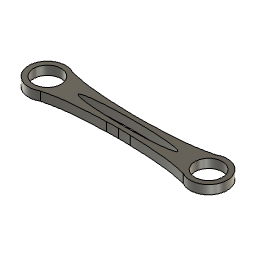
First Arm (Autodesk Fusion 360 design; units mm, degrees)
Autodesk Fusion 360 part; units mm, degrees
note: some values were not read from the file. Set by a fixed rule: which sketch regions a step uses.
sketch "Sketch1" plane through (0, 0, 0) normal (0, 0, 1) x (1, 0, 0)
  circle A0 centre (0, 0) radius 11.0625
  circle A1 centre (0, 0) radius 15
  line L0 (0, 0) -> (130, 0)
  circle A2 centre (130, 0) radius 11.0625
  circle A3 centre (130, 0) radius 15
  line L1 (0, 0) -> (65, 0)
  spline S0 degree 5 poles (7.4528, 13.0175) (7.8836, 12.9141) (8.7411, 12.7102) (10.015, 12.4132) (11.688, 12.0352) (13.7317, 11.594) (15.7226, 11.1861) (17.6579, 10.8135) (19.5392, 10.4779) (21.3761, 10.1803) (23.1841, 9.9205) (24.9799, 9.6971) (26.7778, 9.5065) (28.5855, 9.3432) (30.3994, 9.1985) (32.2092, 9.0627) (34.0044, 8.9273) (35.7794, 8.7866) (37.5401, 8.6406) (39.3083, 8.496) (41.1126, 8.3625) (42.9802, 8.2492) (44.9302, 8.1618) (46.9629, 8.0975) (49.0581, 8.0448) (51.1857, 7.988) (52.8875, 7.9263) (54.152, 7.865) (54.9881, 7.8168) (55.4044, 7.7909) knots 0 0 0 0 0 0 0.04 0.08 0.12 0.16 0.2 0.24 0.28 0.32 0.36 0.4 0.44 0.48 0.52 0.56 0.6 0.64 0.68 0.72 0.76 0.8 0.84 0.88 0.92 0.96 1 1 1 1 1 1
  line L2 (65, 0) -> (65, 43.1808)
  spline S1 degree 5 poles (55.4044, 7.7909) (55.7874, 7.7593) (56.5538, 7.7035) (57.7049, 7.642) (59.2419, 7.5975) (61.1644, 7.58) (62.701, 7.5793) (63.8515, 7.5799) (64.6173, 7.5801) (65, 7.5801) knots 0 0 0 0 0 0 0.2 0.4 0.6 0.8 1 1 1 1 1 1
  spline S2 degree 5 poles (122.5472, 13.0175) (122.1164, 12.9141) (121.2589, 12.7102) (119.985, 12.4132) (118.312, 12.0352) (116.2683, 11.594) (114.2774, 11.1861) (112.3421, 10.8135) (110.4608, 10.4779) (108.6239, 10.1803) (106.8159, 9.9205) (105.0201, 9.6971) (103.2222, 9.5065) (101.4145, 9.3432) (99.6006, 9.1985) (97.7908, 9.0627) (95.9956, 8.9273) (94.2206, 8.7866) (92.4599, 8.6406) (90.6917, 8.496) (88.8874, 8.3625) (87.0198, 8.2492) (85.0698, 8.1618) (83.0371, 8.0975) (80.9419, 8.0448) (78.8143, 7.988) (77.1125, 7.9263) (75.848, 7.865) (75.0119, 7.8168) (74.5956, 7.7909) knots 0 0 0 0 0 0 0.04 0.08 0.12 0.16 0.2 0.24 0.28 0.32 0.36 0.4 0.44 0.48 0.52 0.56 0.6 0.64 0.68 0.72 0.76 0.8 0.84 0.88 0.92 0.96 1 1 1 1 1 1
  line L3 (2.3089, 14.2524) -> (12.5967, 11.7826)
  line L4 (50.4549, 8.0994) -> (60.354, 7.4823)
  line L5 (127.6911, 14.2524) -> (117.4033, 11.7826)
  line L6 (79.5451, 8.0994) -> (69.646, 7.4823)
  spline S3 degree 5 poles (74.5956, 7.7909) (74.2126, 7.7593) (73.4462, 7.7035) (72.2951, 7.642) (70.7581, 7.5975) (68.8356, 7.58) (67.299, 7.5793) (66.1485, 7.5799) (65.3827, 7.5801) (65, 7.5801) knots 0 0 0 0 0 0 0.2 0.4 0.6 0.8 1 1 1 1 1 1
  line L7 (54.4257, 7.8715) -> (56.3832, 7.7102)
  line L8 (64.0213, 7.5801) -> (65.9787, 7.5801)
  line L9 (75.5743, 7.8715) -> (73.6168, 7.7102)
  line L10 (65.9787, 7.5801) -> (64.0213, 7.5801)
  spline S4 degree 5 poles (122.5472, -13.0175) (122.1164, -12.9141) (121.2589, -12.7102) (119.985, -12.4132) (118.312, -12.0352) (116.2683, -11.594) (114.2774, -11.1861) (112.3421, -10.8135) (110.4608, -10.4779) (108.6239, -10.1803) (106.8159, -9.9205) (105.0201, -9.6971) (103.2222, -9.5065) (101.4145, -9.3432) (99.6006, -9.1985) (97.7908, -9.0627) (95.9956, -8.9273) (94.2206, -8.7866) (92.4599, -8.6406) (90.6917, -8.496) (88.8874, -8.3625) (87.0198, -8.2492) (85.0698, -8.1618) (83.0371, -8.0975) (80.9419, -8.0448) (78.8143, -7.988) (77.1125, -7.9263) (75.848, -7.865) (75.0119, -7.8168) (74.5956, -7.7909) knots 0 0 0 0 0 0 0.04 0.08 0.12 0.16 0.2 0.24 0.28 0.32 0.36 0.4 0.44 0.48 0.52 0.56 0.6 0.64 0.68 0.72 0.76 0.8 0.84 0.88 0.92 0.96 1 1 1 1 1 1
  line L11 (127.6911, -14.2524) -> (117.4033, -11.7826)
  line L12 (79.5451, -8.0994) -> (69.646, -7.4823)
  spline S5 degree 5 poles (74.5956, -7.7909) (74.2126, -7.7593) (73.4462, -7.7035) (72.2951, -7.642) (70.7581, -7.5975) (68.8356, -7.58) (67.299, -7.5793) (66.1485, -7.5799) (65.3827, -7.5801) (65, -7.5801) knots 0 0 0 0 0 0 0.2 0.4 0.6 0.8 1 1 1 1 1 1
  line L13 (75.5743, -7.8715) -> (73.6168, -7.7102)
  line L14 (65.9787, -7.5801) -> (64.0213, -7.5801)
  spline S6 degree 5 poles (55.4044, -7.7909) (55.7874, -7.7593) (56.5538, -7.7035) (57.7049, -7.642) (59.2419, -7.5975) (61.1644, -7.58) (62.701, -7.5793) (63.8515, -7.5799) (64.6173, -7.5801) (65, -7.5801) knots 0 0 0 0 0 0 0.2 0.4 0.6 0.8 1 1 1 1 1 1
  line L15 (54.4257, -7.8715) -> (56.3832, -7.7102)
  line L16 (64.0213, -7.5801) -> (65.9787, -7.5801)
  spline S7 degree 5 poles (7.4528, -13.0175) (7.8836, -12.9141) (8.7411, -12.7102) (10.015, -12.4132) (11.688, -12.0352) (13.7317, -11.594) (15.7226, -11.1861) (17.6579, -10.8135) (19.5392, -10.4779) (21.3761, -10.1803) (23.1841, -9.9205) (24.9799, -9.6971) (26.7778, -9.5065) (28.5855, -9.3432) (30.3994, -9.1985) (32.2092, -9.0627) (34.0044, -8.9273) (35.7794, -8.7866) (37.5401, -8.6406) (39.3083, -8.496) (41.1126, -8.3625) (42.9802, -8.2492) (44.9302, -8.1618) (46.9629, -8.0975) (49.0581, -8.0448) (51.1857, -7.988) (52.8875, -7.9263) (54.152, -7.865) (54.9881, -7.8168) (55.4044, -7.7909) knots 0 0 0 0 0 0 0.04 0.08 0.12 0.16 0.2 0.24 0.28 0.32 0.36 0.4 0.44 0.48 0.52 0.56 0.6 0.64 0.68 0.72 0.76 0.8 0.84 0.88 0.92 0.96 1 1 1 1 1 1
  line L17 (2.3089, -14.2524) -> (12.5967, -11.7826)
  line L18 (50.4549, -8.0994) -> (60.354, -7.4823)
  ellipse E0 centre (65, 0) end of major axis (25, 0) minor radius 4
  line L19 (105, 0) -> (25, 0) construction
  line L20 (65, 4) -> (65, -4) construction
  point P0 (18.3178, 10.6996)
  point P1 (27.044, 9.4876)
  point P2 (35.5289, 8.8053)
  point P3 (44.207, 8.1979)
  point P4 (111.6822, 10.6996)
  point P5 (102.956, 9.4876)
  point P6 (94.4711, 8.8053)
  point P7 (85.793, 8.1979)
  point P8 (111.6822, -10.6996)
  point P9 (102.956, -9.4876)
  point P10 (94.4711, -8.8053)
  point P11 (85.793, -8.1979)
  point P12 (18.3178, -10.6996)
  point P13 (27.044, -9.4876)
  point P14 (35.5289, -8.8053)
  point P15 (44.207, -8.1979)
  dimension "d1" = 22.125
  dimension "d2" = 30
  dimension "d3" = 130
  dimension "d4" = 22.125
  dimension "d5" = 30
  dimension "d6" = 65
  constraint coincident A0.centre A1.centre
  constraint concentric A0 A1
  constraint horizontal L0
  constraint coincident L0.end A2.centre
  constraint concentric A2 A3
  constraint parallel L0 L1
  constraint coincident A1 S0.start
  constraint perpendicular L1 L2
  constraint coincident L2 S1.end
  constraint midpoint S0.start L3
  constraint midpoint S0.end L4
  constraint midpoint S0.end L7
  constraint midpoint S1.end L8
  constraint symmetric S0.start L2 S2.start
  constraint symmetric P0 L2 P4
  constraint symmetric P1 L2 P5
  constraint symmetric P2 L2 P6
  constraint symmetric P3 L2 P7
  constraint symmetric S0.end L2 S2.end
  constraint symmetric L2 L3.start L5.start
  constraint symmetric L2 L3.end L5.end
  constraint symmetric L2 L4.start L6.start
  constraint symmetric L2 L4.end L6.end
  constraint symmetric L2 L7.start L9.start
  constraint symmetric L2 L7.end L9.end
  constraint symmetric L2 L8.start L8.end
  constraint symmetric L2 L8.end L8.start
  constraint coincident L8.start L10.end
  constraint symmetric L0 S0.start S7.start
  constraint symmetric L0 P0 P12
  constraint symmetric L0 P1 P13
  constraint symmetric L0 P2 P14
  constraint symmetric L0 P3 P15
  constraint symmetric L0 S0.end S6.start
  constraint symmetric L0 S1.end S5.end
  constraint symmetric L0 S2.start S4.start
  constraint symmetric L0 P4 P8
  constraint symmetric L0 P5 P9
  constraint symmetric L0 P6 P10
  constraint symmetric L0 P7 P11
  constraint symmetric L0 S2.end S4.end
  constraint symmetric L0 L3.start L17.start
  constraint symmetric L0 L3.end L17.end
  constraint symmetric L0 L4.start L18.start
  constraint symmetric L0 L4.end L18.end
  constraint symmetric L0 L5.start L11.start
  constraint symmetric L0 L5.end L11.end
  constraint symmetric L0 L6.start L12.start
  constraint symmetric L0 L6.end L12.end
  constraint symmetric L0 L7.start L15.start
  constraint symmetric L0 L7.end L15.end
  constraint symmetric L0 L8.start L14.end
  constraint symmetric L0 L8.end L14.start
  constraint symmetric L0 L9.start L13.start
  constraint symmetric L0 L9.end L13.end
  constraint coincident E0 L19.start
  constraint coincident E0 L19.end
  constraint coincident E0 L20.start
  constraint coincident E0 L20.end
  constraint coincident L1.end L2.start
  constraint perpendicular L2 L19
  measures "d1" diameter of A0
  measures "d2" diameter of A1
  measures "d3" distance of A0.centre L0.end
  measures "d4" diameter of A2
  measures "d5" diameter of A3
  measures "d6" distance of A0.centre L1.end
extrude "Extrude1" add sketch "Sketch1" along normal blind 7.142 contours A1 | A1 L0 A3 L1 S4 S5 L14 S6 L16 S7 E0 | A1 L0 L1 S0 L2 S1 L8 L10 E0 | L0 A3 L2 S2 S3 L8 L10 E0 | A3
